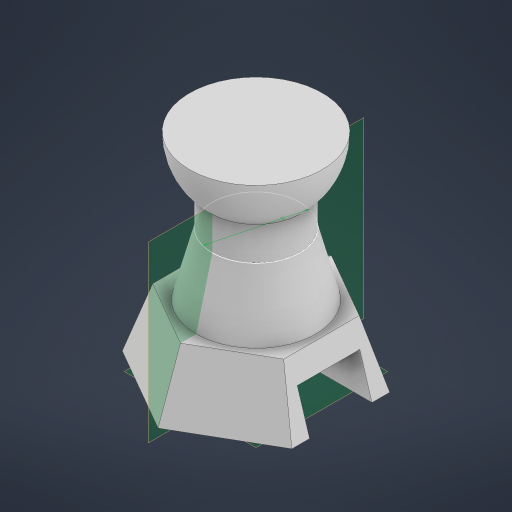
# Autodesk Inventor part: PartE
Saved by Autodesk Inventor 2024.3 (Build 283343000, 343)
## iProperties
Created: 2025-07-08
Part Number: PartE
Material: Generic
Document SubType Name: Modeling
Designer: LeoFB
Density: 1 g/cm^3
Appearance: Default
Author: LeoFB
Autodesk Inventor part; units mm, degrees
ref_plane "YZ Plane" through (0, 0, 0) normal (1, 0, 0) x (0, 1, 0)
ref_plane "XZ Plane" through (0, 0, 0) normal (0, 1, 0) x (-1, 0, 0)
ref_plane "XY Plane" through (0, 0, 0) normal (0, 0, 1) x (1, 0, 0)
sketch "Sketch2" plane through (0, 0, 0) normal (0, 1, 0) x (-1, 0, 0)
  circle A0 centre (0, 0) radius 21
  dimension "d1" = 42
  constraints: 1 centre point, 1 coincident
  measures "d1" diameter of A0
extrude "Extrusion1" add sketch "Sketch2" along normal mid plane 16
sketch "Sketch3" plane through (0, -8, 0) normal (0, -1, 0) x (1, 0, 0)
  circle A0 centre (0, 0) radius 21
  dimension "d4" = 42
  constraints: 1 centre point, 1 coincident
  measures "d4" diameter of A0
ref_plane "Work Plane1" through (0, -38, 0) normal (0, -1, 0) x (1, 0, 0)
sketch "Sketch4" plane through (0, -38, 0) normal (0, -1, 0) x (1, 0, 0)
  circle A0 centre (0, 0) radius 28.77
  dimension "d6" = 57.54
  constraints: 1 centre point, 1 coincident
  measures "d6" diameter of A0
loft "Loft1" add profiles "Sketch4" section 1 edges at (21, -8, 0)
sketch "Sketch5" plane through (0, -38, 0) normal (0, -1, 0) x (1, 0, 0)
  circle A0 centre (0, 0) radius 28.77 projected
  line L0 (0, 0) -> (28.77, 0) construction
  line L1 (0, 36.3025) -> (31.4389, 18.1512)
  line L2 (31.4389, 18.1512) -> (31.4389, -18.1512)
  line L3 (31.4389, -18.1512) -> (0, -36.3025)
  line L4 (0, -36.3025) -> (-31.4389, -18.1512)
  line L5 (-31.4389, -18.1512) -> (-31.4389, 18.1512)
  line L6 (-31.4389, 18.1512) -> (0, 36.3025)
  constraints: 14 end point, 2 coincident, 1 horizontal, 13 other
ref_plane "Work Plane2" through (0, -68, 0) normal (0, -1, 0) x (1, 0, 0)
sketch "Sketch6" plane through (0, -38, 0) normal (0, -1, 0) x (1, 0, 0)
  point P0 (0, 0)
sketch "Sketch8" plane through (0, -68, 0) normal (0, -1, 0) x (1, 0, 0)
  line L0 (0, 47.0378) -> (40.7359, 23.5189)
  line L1 (40.7359, 23.5189) -> (40.7359, -23.5189)
  line L2 (40.7359, -23.5189) -> (0, -47.0378)
  line L3 (0, -47.0378) -> (-40.7359, -23.5189)
  line L4 (-40.7359, -23.5189) -> (-40.7359, 23.5189)
  line L5 (-40.7359, 23.5189) -> (0, 47.0378)
  point P0 (0, 0)
  point P1 (0, 0)
  constraints: 12 end point, 1 coincident, 13 other
loft "Loft3" add profiles "Sketch8", "Sketch5" contours all / A0 | L1 L2 L3 L4 L5 L6
sketch "Sketch9" plane through (-40.7359, -68, -23.5189) normal (-0.9551836, 0.296014, 0) x (0, 0, 1)
  line L0 (0, 0) -> (47.0378, 0) projected
  line L1 (23.5189, 0) -> (16.0189, 0)
  line L2 (31.0189, 0) -> (23.5189, 0)
  line L3 (31.0189, 0) -> (16.0189, 0)
  line L4 (16.0189, 20) -> (31.0189, 20)
  line L5 (23.5189, 0) -> (8.5189, 0)
  line L6 (8.5189, 0) -> (8.5189, 20)
  line L7 (8.5189, 20) -> (38.5189, 20)
  line L8 (38.5189, 20) -> (38.5189, 0)
  point P0 (23.5189, 77.0109)
  dimension "d40" = 15
  dimension "d41" = 20
  dimension "d42" = 30
  constraints: 16 end point, 3 perpendicular, 2 horizontal, 2 point on line, 1 midpoint, 1 parallel
  measures "d40" distance of L2.end L5.end
  measures "d41" distance of L5.end L6.end
  measures "d42" distance of L6.end L7.end
sketch "Sketch10" plane through (40.7359, -68, 23.5189) normal (0.9551836, 0.296014, 0) x (0, 0, -1)
  line L0 (38.5189, 20) -> (38.5189, 0)
  line L1 (8.5189, 0) -> (8.5189, 20)
  line L2 (8.5189, 20) -> (38.5189, 20)
  line L3 (38.5189, 20) -> (38.5189, 0)
  line L4 (0, 0) -> (47.0378, 0) projected
  line L5 (8.5189, 0) -> (38.5189, 0)
  point P0 (23.5189, 77.0109)
  point P1 (23.5189, 0)
  point P2 (53.5189, 0)
  point P3 (23.5189, 0)
  constraints: 10 end point, 2 point on line, 1 parallel
loft "Loft4" cut profiles "Sketch9", "Sketch10"
ref_plane "Work Plane4" through (0, 63.4475, -18.1512) normal (-1, 0, 0) x (0, 0, 1)
sketch "Sketch12" plane through (0, 63.4475, -18.1512) normal (-1, 0, 0) x (0, 0, 1)
  line L0 (39.1512, -55.4475) -> (-2.8488, -55.4475) projected
  line L1 (18.1512, -55.4475) -> (39.1512, -55.4475)
  arc A0 (39.1512, -55.4475) -> (50.0417, -31.4475) centre (18.1512, -31.4475) ccw
  line L2 (18.1512, -31.4475) -> (50.0417, -31.4475)
  line L3 (18.1512, -31.4475) -> (18.1512, -55.4475)
  line L4 (18.1512, -55.4475) -> (39.1512, -55.4475)
  point P0 (18.1512, -63.4475)
  constraints: 9 end point, 2 point on circle, 1 centre point, 1 collinear, 1 horizontal, 1 midpoint, 1 perpendicular
revolve "Revolution1" add sketch "Sketch12" angle 360 about axis through (0, 32, 0) along (0, -1, 0)
body "Solid1"
